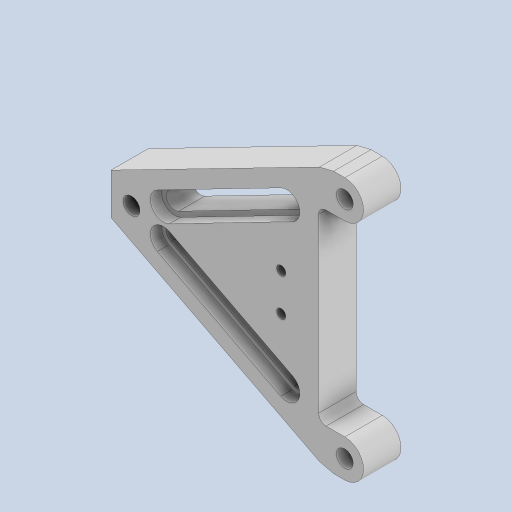
# Autodesk Inventor part: V structure
Saved by Autodesk Inventor 2023.4 (Build 274418000, 418)
## iProperties
Created: 2023-12-14
Part Number: V structure
Material: Generic
Document SubType Name: Modeling
Designer: PalumaCMM
Density: 1 g/cm^3
Appearance: Default
Author: PalumaCMM
Autodesk Inventor part; units mm, degrees
ref_plane "YZ Plane" through (0, 0, 0) normal (1, 0, 0) x (0, 1, 0)
ref_plane "XZ Plane" through (0, 0, 0) normal (0, 1, 0) x (-1, 0, 0)
ref_plane "XY Plane" through (0, 0, 0) normal (0, 0, 1) x (1, 0, 0)
sketch "Sketch1" plane through (0, 0, 0) normal (0, 0, 1) x (1, 0, 0)
  arc A0 (2.25, 0) -> (-2.25, 0) centre (0, 0) ccw
  line L0 (0, 0) -> (-2.25, 0) construction
  line L1 (0, 0) -> (2.25, 0) construction
  line L2 (5.5, 0) -> (-5.5, 0)
  line L3 (-5.5, 0) -> (-5.5, 5.5)
  line L4 (-5.5, 5.5) -> (5.5, 5.5)
  line L5 (5.5, 5.5) -> (5.5, 0)
  line L6 (-19, 0) -> (75.5, 0) projected
  circle A1 centre (57, 30) radius 2.25
  circle A2 centre (57, 30) radius 5
  line L7 (-5.5, 5.5) -> (52, 35)
  line L8 (52, 35) -> (57, 35)
  line L9 (57, 25) -> (50, 25)
  line L10 (50, 25) -> (50, 0)
  line L11 (-5.5, 0) -> (50, 0)
  point P0 (52, 30)
  point P1 (-2.25, 0)
  point P2 (50, 0)
  dimension "d0" = 2.25
  dimension "d1" = 180
  dimension "d2" = 11
  dimension "d3" = 5.5
  dimension "d4" = 4.5
  dimension "d5" = 10
  dimension "d6" = 25
  dimension "d7" = 90
  dimension "d8" = 55.5
  dimension "d42" = 64.6258
  dimension "d43" = 5
  constraints: 22 end point, 5 point on circle, 4 horizontal, 3 centre point, 3 coincident, 3 collinear, 2 parallel, 2 perpendicular, 2 tangent
  measures "d0" radius of A0
  measures "d1" angle of L0 L1
  measures "d2" distance of L3.end L4.end
  measures "d3" distance of L2.end L3.end
  measures "d4" diameter of A1
  measures "d5" diameter of A2
  measures "d6" distance of L9.end L10.end
  measures "d7" angle of L10 L9
  measures "d8" distance of L2.end L10.end
  measures "d42" distance of L3.end L7.end
  measures "d43" distance of L7.end L8.end
extrude "Extrusion1" add sketch "Sketch1" along normal blind 10 contours A0 L2 L3 L4 L5 | L5 L4 L7 L8 A2 L9 L10 L6 | A2
mirror "Mirror1" about plane through (0, 0, 0) normal (0, 1, 0)
fillet "Fillet1" radius 2 2 edges at (50, 25, 5) (50, -25, 5)
sketch "Sketch2" plane through (0, 0, 10) normal (0, 0, 1) x (1, 0, 0)
  circle A0 centre (0, 0) radius 2.25 projected
  line L0 (0, 0) -> (69.506, 0)
  line L1 (0, 0) -> (0, 32.0889)
  line L2 (41.5, 21) -> (8.5, 4) construction
  line L3 (40.4696, 23.0002) -> (7.4696, 6.0002)
  line L4 (9.5304, 1.9998) -> (42.5304, 18.9998)
  arc A1 (42.5304, 18.9998) -> (40.4696, 23.0002) centre (41.5, 21) ccw
  arc A2 (7.4696, 6.0002) -> (9.5304, 1.9998) centre (8.5, 4) ccw
  line L5 (41.5, 21) -> (8.5, 4) construction
  line L6 (39.8972, 24.1114) -> (6.8972, 7.1114)
  line L7 (10.1028, 0.8886) -> (43.1028, 17.8886)
  arc A3 (43.1028, 17.8886) -> (39.8972, 24.1114) centre (41.5, 21) ccw
  arc A4 (6.8972, 7.1114) -> (10.1028, 0.8886) centre (8.5, 4) ccw
  arc A5 (52, 25) -> (50, 23) centre (52, 23) ccw construction
  line L8 (52, 25) -> (57, 25) construction
  arc A6 (57, 25) -> (57, 35) centre (57, 30) ccw construction
  line L9 (57, 35) -> (52, 35) construction
  line L10 (52, 35) -> (-5.5, 5.5) construction
  line L11 (-5.5, 5.5) -> (-5.5, -5.5) construction
  line L12 (52, -35) -> (-5.5, -5.5) construction
  line L13 (57, -35) -> (52, -35) construction
  arc A7 (57, -35) -> (57, -25) centre (57, -30) ccw construction
  line L14 (52, -25) -> (57, -25) construction
  arc A8 (50, -23) -> (52, -25) centre (52, -23) ccw construction
  line L15 (50, 23) -> (50, -23) construction
  circle A9 centre (57, -30) radius 2.25 construction
  circle A10 centre (0, 0) radius 2.25 construction
  circle A11 centre (57, 30) radius 2.25 construction
  point P0 (25, 12.5)
  point P1 (25, 12.5)
  dimension "d15" = 4.5
  dimension "d16" = 7
  dimension "d38" = 47
  dimension "d39" = 14
  dimension "d40" = 4
  dimension "d41" = 21
  constraints: 20 end point, 8 point on circle, 8 tangent, 4 centre point, 3 equal length, 2 midpoint, 1 horizontal, 1 vertical
  measures "d15" diameter of A2
  measures "d16" diameter of A4
  measures "d38" distance from line of L11 L2.start
  measures "d39" distance from line of L11 L2.end
  measures "d40" distance from line of L0 L2.end
  measures "d41" vertical distance of point (0, 0) L2.start
extrude "Extrusion2" cut sketch "Sketch2" against normal blind 3 contours A3 L7 A4 L6
sketch "Sketch3" plane through (0, 0, 10) normal (0, 0, 1) x (1, 0, 0)
  arc A0 (42.5304, 18.9998) -> (40.4696, 23.0002) centre (41.5, 21) ccw projected
  arc A1 (7.4696, 6.0002) -> (9.5304, 1.9998) centre (8.5, 4) ccw projected
  line L0 (41.5, 21) -> (8.5, 4) construction
  line L1 (40.4696, 23.0002) -> (7.4696, 6.0002)
  line L2 (9.5304, 1.9998) -> (42.5304, 18.9998)
  arc A2 (42.5304, 18.9998) -> (40.4696, 23.0002) centre (41.5, 21) ccw
  arc A3 (7.4696, 6.0002) -> (9.5304, 1.9998) centre (8.5, 4) ccw
  point P0 (0, 0)
  point P1 (25, 12.5)
  dimension "d19" = 4.5
  constraints: 8 end point, 4 point on circle, 4 tangent, 2 centre point, 1 midpoint, 1 parallel
  measures "d19" diameter of A3
extrude "Extrusion3" cut sketch "Sketch3" against normal blind 10
mirror "Mirror2" about plane through (0, 0, 0) normal (0, 1, 0) of "Extrusion2", "Extrusion1", "Extrusion3"
sketch "Sketch4" plane through (0, 0, 10) normal (0, 0, 1) x (1, 0, 0)
  circle A0 centre (40, 5) radius 1.75
  point P0 (0, 0)
  dimension "d24" = 3.5
  constraints: 1 centre point
  measures "d24" diameter of A0
hole "Hole1" at (40, 5, 10) direction (0, 0, -1) diameter 2.459 end through all thread size "M3x0.5" class "6H" standard "ISO Metric profile"
mirror "Mirror6" about plane through (0, 0, 0) normal (0, 1, 0) of "Hole1", "Extrusion2", "Extrusion3"
chamfer "Chamfer1" distance 2 angle 45 1 edges at (52, 35, 5)
chamfer "Chamfer2" distance 2 angle 45 1 edges at (52, -35, 5)
body "Solid1"
